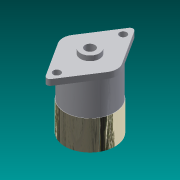
# Autodesk Inventor part: GM15BY_StepMotor
Saved by Autodesk Inventor 2015 (Build 190159000, 159)
## iProperties
Created: 2018-12-01
Part Number: GM15BY_StepMotor
Material: Generic
Document SubType Name: Modeling
Designer: tlsru
Density: 1 g/cm^3
Appearance: 흰색
Author: tlsru
Autodesk Inventor part; units mm, degrees
ref_plane "YZ Plane" through (0, 0, 0) normal (1, 0, 0) x (0, 1, 0)
ref_plane "XZ Plane" through (0, 0, 0) normal (0, 1, 0) x (-1, 0, 0)
ref_plane "XY Plane" through (0, 0, 0) normal (0, 0, 1) x (1, 0, 0)
sketch "스케치1" plane through (0, 0, 0) normal (0, 0, 1) x (1, 0, 0)
  circle A0 centre (0, 0) radius 1.5
  circle A1 centre (0, 0) radius 2.9
  dimension "d0" = 3
  dimension "d1" = 5.8
  constraints: 2 centre point, 2 coincident
  measures "d0" diameter of A0
  measures "d1" diameter of A1
extrude "돌출1" add sketch "스케치1" along normal blind 1.5
sketch "스케치2" plane through (0, 0, 0) normal (0, 0, -1) x (-1, 0, 0)
  line L0 (7.6095, 2.163) -> (0.8412, 12.6915)
  line L1 (-0.8412, 12.6915) -> (-7.6095, 2.163)
  line L2 (7.6095, -2.163) -> (0.8412, -12.6915)
  line L3 (-0.8412, -12.6915) -> (-7.6095, -2.163)
  circle A0 centre (0, 10.1) radius 1.1
  circle A1 centre (0, -10.1) radius 1.1
  arc A2 (0.8412, 12.6915) -> (-0.8412, 12.6915) centre (0, 12.1507) ccw
  arc A3 (-0.8412, -12.6915) -> (0.8412, -12.6915) centre (0, -12.1507) ccw
  arc A4 (7.6095, -2.163) -> (7.6095, 2.163) centre (4.2448, 0) ccw
  arc A5 (-7.6095, 2.163) -> (-7.6095, -2.163) centre (-4.2448, 0) ccw
  circle A6 centre (0, 0) radius 1.5 projected
  dimension "d8" = 2.2
  dimension "d9" = 2.2
  dimension "d10" = 10.1
  dimension "d11" = 10.1
  dimension "d12" = 1
  dimension "d13" = 4
  constraints: 8 end point, 8 point on circle, 8 tangent, 6 centre point, 2 equal radius, 2 parallel
  measures "d8" diameter of A0
  measures "d9" diameter of A1
  measures "d10" distance of point (0, 0) A1.centre
  measures "d11" distance of A0.centre point (0, 0)
  measures "d12" radius of A2
  measures "d13" radius of A4
extrude "돌출2" add sketch "스케치2" along normal blind 1.8
sketch "스케치3" plane through (0, 0, -1.8) normal (0, 0, -1) x (-1, 0, 0)
  circle A0 centre (0, 0) radius 1.5 projected
  circle A1 centre (0, -10.1) radius 1.1 projected
  circle A2 centre (0, 10.1) radius 1.1 projected
  line L0 (-0.8412, 12.6915) -> (-7.6095, 2.163) projected
  arc A3 (-7.6095, 2.163) -> (-7.6095, -2.163) centre (-4.2448, 0) ccw projected
  line L1 (-7.6095, -2.163) -> (-0.8412, -12.6915) projected
  arc A4 (-0.8412, -12.6915) -> (0.8412, -12.6915) centre (0, -12.1507) ccw projected
  line L2 (0.8412, -12.6915) -> (7.6095, -2.163) projected
  arc A5 (7.6095, -2.163) -> (7.6095, 2.163) centre (4.2448, 0) ccw projected
  line L3 (7.6095, 2.163) -> (0.8412, 12.6915) projected
  arc A6 (0.8412, 12.6915) -> (-0.8412, 12.6915) centre (0, 12.1507) ccw projected
  circle A7 centre (0, 0) radius 1.5 projected
  circle A8 centre (0, 0) radius 7.5
  dimension "d16" = 15
  constraints: 1 centre point, 1 coincident
  measures "d16" diameter of A8
extrude "돌출3" add sketch "스케치3" along normal blind 10 contours A0 | A8
sketch "스케치4" plane through (0, 0, -11.8) normal (0, 0, -1) x (-1, 0, 0)
  circle A0 centre (0, 0) radius 7.5 projected
  circle A1 centre (0, 0) radius 7.6
  dimension "d19" = 0.1
  constraints: 1 centre point
  measures "d19" radial gap between concentric circles of A0 A1
extrude "돌출4" add sketch "스케치4" along normal blind 9 contours A0 | A1
